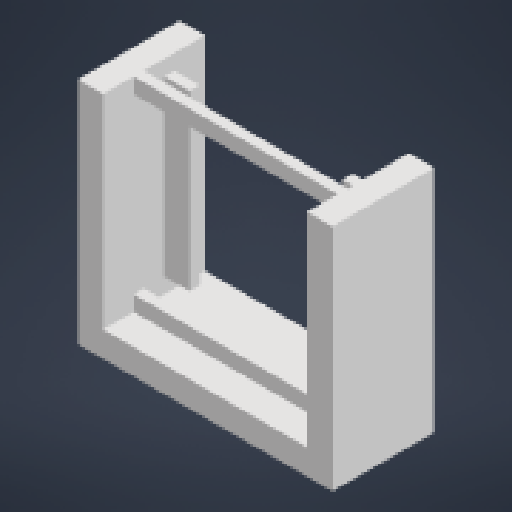
# Autodesk Inventor part: Sensorroom
Saved by Autodesk Inventor 2026.2 (Build 302298000, 298)
## iProperties
Created: 2026-03-10
Part Number: Sensorroom
Material: Generic
Document SubType Name: Modeling
Designer: danda
Density: 1 g/cm^3
Appearance: Default
Author: danda
Autodesk Inventor part; units mm, degrees
ref_plane "YZ Plane" through (0, 0, 0) normal (1, 0, 0) x (0, 1, 0)
ref_plane "XZ Plane" through (0, 0, 0) normal (0, 1, 0) x (-1, 0, 0)
ref_plane "XY Plane" through (0, 0, 0) normal (0, 0, 1) x (1, 0, 0)
sketch "Sketch1" plane through (0, 0, 0) normal (0, 0, 1) x (1, 0, 0)
  line L0 (4.914, 16.1404) -> (44.914, 16.1404)
  line L1 (44.914, 16.1404) -> (44.914, -23.8596)
  line L2 (44.914, -23.8596) -> (4.914, -23.8596)
  line L3 (4.914, -23.8596) -> (4.914, 16.1404)
  line L4 (49.914, 21.1404) -> (-0.086, 21.1404)
  line L5 (-0.086, 21.1404) -> (-0.086, -28.8596)
  line L6 (-0.086, -28.8596) -> (49.914, -28.8596)
  line L7 (49.914, -28.8596) -> (49.914, 21.1404)
  line L8 (4.914, 16.1404) -> (-0.086, 16.1404)
  line L9 (44.914, 16.1404) -> (49.914, 16.1404)
  line L10 (4.914, -20.8596) -> (44.914, -20.8596)
  line L11 (4.914, 13.1404) -> (44.914, 13.1404)
  line L12 (9.914, 13.1404) -> (9.914, -20.8596)
  line L13 (39.914, 13.1404) -> (39.914, -20.8596)
  point P0 (0, 0)
  dimension "d0" = 40
  dimension "d1" = 40
  dimension "d2" = 5
  dimension "d3" = 3
  dimension "d4" = 3
  dimension "d5" = 5
  dimension "d6" = 5
  constraints: 28 end point, 11 point on line, 7 perpendicular, 4 parallel, 1 horizontal, 3 other
  measures "d0" distance of L1.end L2.end
  measures "d1" distance of L0.end L1.end
  measures "d2" distance between parallel lines of L0 L4
  measures "d3" distance between parallel lines of L2 L10
  measures "d4" distance between parallel lines of L11 L0
  measures "d5" distance between parallel lines of L13 L1
  measures "d6" distance between parallel lines of L3 L12
extrude "Extrusion1" add sketch "Sketch1" along normal mid plane 20 contours L3 L2 L1 L9 L7 L6 L5 L8
extrude "Extrusion2" add sketch "Sketch1" along normal blind 4 contours L0 L1 L11 L3 | L10 L1 L2 L3
extrude "Extrusion3" cut sketch "Sketch1" along normal blind 2 contours L0 L1 L11 L3 | L10 L1 L2 L3
extrude "Extrusion4" add sketch "Sketch1" against normal blind 4 contours L11 L12 L10 L3 | L1 L10 L13 L11
extrude "Extrusion5" cut sketch "Sketch1" against normal blind 2 contours L11 L12 L10 L3 | L1 L10 L13 L11
body "Solid1"
